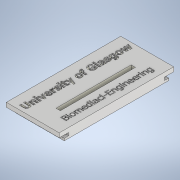
# Autodesk Inventor part: top
Saved by Autodesk Inventor 2021 (Build 250183000, 183)
## iProperties
Created: 2019-01-23
Part Number: top
Material: 常规
Document SubType Name: Modeling
Designer: Guo Xin
Density: 1 g/cm^3
Appearance: 默认
Author: Guo Xin
Autodesk Inventor part; units mm, degrees
(part 1 of 2)
ref_plane "YZ Plane" through (0, 0, 0) normal (1, 0, 0) x (0, 1, 0)
ref_plane "XZ Plane" through (0, 0, 0) normal (0, 1, 0) x (-1, 0, 0)
ref_plane "XY Plane" through (0, 0, 0) normal (0, 0, 1) x (1, 0, 0)
sketch "草图1" plane through (0, 0, 0) normal (0, 1, 0) x (-1, 0, 0)
  line L0 (0, 0) -> (37, 0)
  line L1 (37, 0) -> (37, -80)
  line L2 (37, -80) -> (0, -80)
  line L3 (0, -80) -> (0, 0)
  dimension "d0" = 80
  dimension "d1" = 37
  constraints: 8 end point, 2 parallel, 1 horizontal, 1 perpendicular
  measures "d0" distance between parallel lines of L2 L0
  measures "d1" distance between parallel lines of L3 L1
extrude "拉伸1" add sketch "草图1" along normal mid plane 4
sketch "草图2" plane through (0, -2, 0) normal (1, 0, 0) x (0, 0, -1)
  line L0 (0, 3) -> (6.5, 3)
  line L1 (6.5, 3) -> (6.5, 1)
  line L2 (6.5, 1) -> (0, 1)
  line L3 (0, 1) -> (0, 3)
  line L4 (73.5, 3) -> (80, 3)
  line L5 (80, 3) -> (80, 1)
  line L6 (80, 1) -> (73.5, 1)
  line L7 (73.5, 1) -> (73.5, 3)
  line L8 (0, 2) -> (0, 4) projected
  line L9 (80, 4) -> (80, 0) projected
  line L10 (0, 4) -> (80, 4) projected
  dimension "d4" = 6.5
  dimension "d5" = 1
  dimension "d6" = 2
  dimension "d7" = 6.5
  dimension "d8" = 1
  dimension "d9" = 2
  constraints: 16 end point, 4 parallel, 2 collinear, 2 horizontal, 2 perpendicular, 2 point on line
  measures "d4" distance between parallel lines of L5 L7
  measures "d5" distance between parallel lines of L10 L4
  measures "d6" distance between parallel lines of L4 L6
  measures "d7" distance between parallel lines of L1 L3
  measures "d8" distance between parallel lines of L10 L0
  measures "d9" distance between parallel lines of L2 L0
extrude "拉伸2" cut sketch "草图2" against normal blind 80
sketch "草图3" plane through (0, -1, -6.5) normal (0, 0, 1) x (1, 0, 0)
  line L0 (-37, 2) -> (-31.5, 2)
  line L1 (-31.5, 2) -> (-31.5, 0)
  line L2 (-31.5, 0) -> (-37, 0)
  line L3 (-37, 0) -> (-37, 2)
  line L4 (-37, 0) -> (-37, 2) projected
  line L5 (-37, 2) -> (0, 2) projected
  line L6 (0, 0) -> (-37, 0) projected
  point P0 (0, 1)
  dimension "d12" = 5.5
  constraints: 8 end point, 3 collinear, 2 parallel, 1 horizontal, 1 perpendicular
  measures "d12" distance between parallel lines of L1 L3
extrude "拉伸3" cut sketch "草图3" against normal blind 80
sketch "草图4" plane through (0, -2, 0) normal (1, 0, 0) x (0, 0, -1)
  line L0 (0, 1) -> (3.5, 1)
  line L1 (3.5, 1) -> (3.5, 0)
  line L2 (3.5, 0) -> (0, 0)
  line L3 (0, 0) -> (0, 1)
  line L4 (0, 2) -> (0, 1) projected
  line L5 (6.5, 1) -> (0, 1) projected
  line L6 (80, 0) -> (0, 0) projected
  line L7 (76.5, 1) -> (80, 1)
  line L8 (80, 1) -> (80, 0)
  line L9 (80, 0) -> (76.5, 0)
  line L10 (76.5, 0) -> (76.5, 1)
  line L11 (80, 1) -> (80, 0) projected
  line L12 (80, 1) -> (73.5, 1) projected
  dimension "d15" = 3.5
  dimension "d16" = 3.5
  constraints: 16 end point, 4 collinear, 4 horizontal, 4 parallel, 2 perpendicular, 1 other
  measures "d15" distance between parallel lines of L3 L1
  measures "d16" distance between parallel lines of L8 L10
extrude "拉伸4" cut sketch "草图4" against normal blind 80
sketch "草图8" plane through (0, -2, 0) normal (0, -1, 0) x (1, 0, 0)
  line L0 (-37, -76.5) -> (-34, -76.5)
  line L1 (-34, -76.5) -> (-34, -3.5)
  line L2 (-34, -3.5) -> (-37, -3.5)
  line L3 (-37, -3.5) -> (-37, -76.5)
  line L4 (-37, -3.5) -> (-37, -76.5) projected
  line L5 (-37, -76.5) -> (0, -76.5) projected
  line L6 (0, -3.5) -> (-37, -3.5) projected
  point P0 (0, 0)
  dimension "d29" = 3
  constraints: 8 end point, 3 collinear, 2 parallel, 1 horizontal, 1 perpendicular
  measures "d29" distance between parallel lines of L1 L3
extrude "拉伸6" cut sketch "草图8" against normal blind 1
sketch "草图9" plane through (0, 2, 0) normal (0, 1, 0) x (1, 0, 0)
  line L0 (0, 80) -> (-37, 80)
  line L1 (-37, 80) -> (-37, 0)
  line L2 (-37, 0) -> (0, 0)
  line L3 (0, 0) -> (0, 80)
  line L4 (-37, 0) -> (0, 0) projected
  line L5 (0, 0) -> (0, 80) projected
  line L6 (0, 80) -> (-37, 80) projected
  line L7 (-37, 80) -> (-37, 0) projected
  constraints: 8 end point, 4 collinear, 2 parallel, 1 horizontal, 1 perpendicular
extrude "拉伸7" add sketch "草图9" along normal blind 2
sketch "草图10" plane through (0, -2, 0) normal (0, -1, 0) x (1, 0, 0)
  line L0 (-34, -3.5) -> (0, -3.5)
  line L1 (0, -3.5) -> (0, -76.5)
  line L2 (0, -76.5) -> (-34, -76.5)
  line L3 (-34, -76.5) -> (-34, -3.5)
  line L4 (0, -76.5) -> (0, -3.5) projected
  line L5 (0, -3.5) -> (-34, -3.5) projected
  line L6 (-34, -76.5) -> (0, -76.5) projected
  line L7 (-34, -3.5) -> (-34, -76.5) projected
  point P0 (0, 0)
  constraints: 8 end point, 4 collinear, 2 parallel, 1 horizontal, 1 perpendicular
extrude "拉伸8" add sketch "草图10" along normal blind 0.6
sketch "草图5" plane through (0, 2, 0) normal (0, 1, 0) x (1, 0, 0)
  line L0 (-16, 13.75) -> (-13, 13.75)
  line L1 (-13, 13.75) -> (-13, 66.25)
  line L2 (-13, 66.25) -> (-16, 66.25)
  line L3 (-16, 66.25) -> (-16, 13.75)
  line L4 (-37, 80) -> (-37, 0) projected
  line L5 (-37, 0) -> (0, 0) projected
  dimension "d19" = 21
  dimension "d20" = 3
  dimension "d21" = 52.5
  dimension "d22" = 13.75
  constraints: 8 end point, 2 parallel, 1 horizontal, 1 perpendicular
  measures "d19" distance between parallel lines of L3 L4
  measures "d20" distance between parallel lines of L3 L1
  measures "d21" distance between parallel lines of L2 L0
  measures "d22" distance between parallel lines of L5 L0
extrude "拉伸5" cut sketch "草图5" against normal blind 80 and the other way blind 40
sketch "草图12" plane through (0, 4, 0) normal (0, 1, 0) x (1, 0, 0)
  line L0 (-30.9955, 2.3359) -> (-30.9955, 87.8984) construction
  line L1 (-30.9955, 87.8984) -> (-2.4855, 87.8984) construction
  line L2 (-2.4855, 87.8984) -> (-2.4855, 2.3359) construction
  line L3 (-2.4855, 2.3359) -> (-30.9955, 2.3359) construction
  line L4 (-9.1049, 9.2608) -> (-9.1049, 16.3764) construction
  line L5 (-9.1049, 16.3764) -> (47.4861, 16.3764) construction
  line L6 (47.4861, 16.3764) -> (47.4861, 9.2608) construction
  line L7 (47.4861, 9.2608) -> (-9.1049, 9.2608) construction
  spline S0 degree 2 poles (-25.6349, 4.8765) (-25.6349, 3.8676) (-26.6074, 2.7817) (-27.5474, 2.7817) knots 0 0 0 1 2 2 2
  line L8 (-27.5474, 2.7817) -> (-30.7403, 2.7817)
  line L9 (-30.7403, 2.7817) -> (-30.7403, 4.0377)
  line L10 (-30.7403, 4.0377) -> (-27.6203, 4.0377)
  spline S1 degree 2 poles (-27.6203, 4.0377) (-27.0976, 4.0377) (-26.5871, 4.4308) (-26.5871, 4.8765) knots 0 0 0 1 2 2 2
  spline S2 degree 2 poles (-26.5871, 4.8765) (-26.5871, 5.31) (-27.0774, 5.7152) (-27.6203, 5.7152) knots 0 0 0 1 2 2 2
  line L11 (-27.6203, 5.7152) -> (-30.7403, 5.7152)
  line L12 (-30.7403, 5.7152) -> (-30.7403, 6.9713)
  line L13 (-30.7403, 6.9713) -> (-27.5515, 6.9713)
  spline S3 degree 2 poles (-27.5515, 6.9713) (-26.6276, 6.9713) (-25.6349, 5.9137) (-25.6349, 4.8765) knots 0 0 0 1 2 2 2
  line L14 (-25.7403, 11.3959) -> (-25.7403, 10.2128)
  line L15 (-25.7403, 10.2128) -> (-27.6082, 10.2128)
  spline S4 degree 2 poles (-27.6082, 10.2128) (-27.8391, 10.2128) (-28.2929, 10.1763) (-28.3983, 10.1277) knots 0 0 0 1 2 2 2
  spline S5 degree 2 poles (-28.3983, 10.1277) (-28.5279, 10.0669) (-28.6374, 9.84) (-28.6374, 9.6455) knots 0 0 0 1 2 2 2
  spline S6 degree 2 poles (-28.6374, 9.6455) (-28.6374, 9.5037) (-28.5279, 9.2079) (-28.4104, 9.0418) knots 0 0 0 1 2 2 2
  line L16 (-28.4104, 9.0418) -> (-25.7403, 9.0418)
  line L17 (-25.7403, 9.0418) -> (-25.7403, 7.8667)
  line L18 (-25.7403, 7.8667) -> (-29.5126, 7.8667)
  line L19 (-29.5126, 7.8667) -> (-29.5126, 9.0418)
  line L20 (-29.5126, 9.0418) -> (-29.0952, 9.0418)
  spline S7 degree 2 poles (-29.0952, 9.0418) (-29.3383, 9.3295) (-29.6138, 9.8765) (-29.6138, 10.2087) knots 0 0 0 1 2 2 2
  spline S8 degree 2 poles (-29.6138, 10.2087) (-29.6138, 10.7841) (-28.8845, 11.3959) (-28.1957, 11.3959) knots 0 0 0 1 2 2 2
  line L21 (-28.1957, 11.3959) -> (-25.7403, 11.3959)
  line L22 (-25.7403, 13.4421) -> (-25.7403, 12.2671)
  line L23 (-25.7403, 12.2671) -> (-29.5126, 12.2671)
  line L24 (-29.5126, 12.2671) -> (-29.5126, 13.4421)
  line L25 (-29.5126, 13.4421) -> (-25.7403, 13.4421)
  line L26 (-30.0515, 13.4786) -> (-30.0515, 12.2346)
  line L27 (-30.0515, 12.2346) -> (-30.9672, 12.2346)
  line L28 (-30.9672, 12.2346) -> (-30.9672, 13.4786)
  line L29 (-30.9672, 13.4786) -> (-30.0515, 13.4786)
  line L30 (-29.5126, 17.8708) -> (-25.7403, 16.5175)
  line L31 (-25.7403, 16.5175) -> (-25.7403, 15.233)
  line L32 (-25.7403, 15.233) -> (-29.5126, 13.8919)
  line L33 (-29.5126, 13.8919) -> (-29.5126, 15.1277)
  line L34 (-29.5126, 15.1277) -> (-27.0207, 15.8975)
  line L35 (-27.0207, 15.8975) -> (-29.5126, 16.6593)
  line L36 (-29.5126, 16.6593) -> (-29.5126, 17.8708)
  spline S9 degree 2 poles (-25.639, 20.2533) (-25.639, 19.1836) (-26.66, 18.045) (-27.6041, 18.045) knots 0 0 0 1 2 2 2
  spline S10 degree 2 poles (-27.6041, 18.045) (-28.5279, 18.045) (-29.6301, 19.1066) (-29.6301, 20.0629) knots 0 0 0 1 2 2 2
  spline S11 degree 2 poles (-29.6301, 20.0629) (-29.6301, 20.9259) (-28.6941, 21.8011) (-27.827, 21.8011) knots 0 0 0 1 2 2 2
  line L37 (-27.827, 21.8011) -> (-27.4015, 21.8011)
  line L38 (-27.4015, 21.8011) -> (-27.4015, 19.2201)
  spline S12 degree 2 poles (-27.4015, 19.2201) (-27.1382, 19.2363) (-26.7897, 19.4267) (-26.6844, 19.5807) knots 0 0 0 1 2 2 2
  spline S13 degree 2 poles (-26.6844, 19.5807) (-26.579, 19.7306) (-26.4899, 20.1358) (-26.4899, 20.3748) knots 0 0 0 1 2 2 2
  spline S14 degree 2 poles (-26.4899, 20.3748) (-26.4899, 20.5774) (-26.579, 20.9745) (-26.656, 21.1406) knots 0 0 0 1 2 2 2
  spline S15 degree 2 poles (-26.656, 21.1406) (-26.7168, 21.2865) (-26.8667, 21.5296) (-26.9234, 21.6066) knots 0 0 0 1 2 2 2
  line L39 (-26.9234, 21.6066) -> (-26.9234, 21.7322)
  line L40 (-26.9234, 21.7322) -> (-25.951, 21.7322)
  spline S16 degree 2 poles (-25.951, 21.7322) (-25.8942, 21.5864) (-25.797, 21.3513) (-25.7484, 21.1406) knots 0 0 0 1 2 2 2
  spline S17 degree 2 poles (-25.7484, 21.1406) (-25.6957, 20.9502) (-25.639, 20.545) (-25.639, 20.2533) knots 0 0 0 1 2 2 2
  spline S18 degree 2 poles (-28.1106, 20.6423) (-28.4834, 20.6342) (-28.8764, 20.306) (-28.8764, 19.9697) knots 0 0 0 1 2 2 2
  spline S19 degree 2 poles (-28.8764, 19.9697) (-28.8764, 19.6252) (-28.4631, 19.2363) (-28.1106, 19.216) knots 0 0 0 1 2 2 2
  line L41 (-28.1106, 19.216) -> (-28.1106, 20.6423)
  line L42 (-28.3983, 24.9372) -> (-28.3983, 24.84)
  spline S20 degree 2 poles (-28.3983, 24.84) (-28.4226, 24.7711) (-28.4469, 24.5158) (-28.4469, 24.3619) knots 0 0 0 1 2 2 2
  spline S21 degree 2 poles (-28.4469, 24.3619) (-28.4469, 24.1795) (-28.3375, 23.7703) (-28.2646, 23.5799) knots 0 0 0 1 2 2 2
  line L43 (-28.2646, 23.5799) -> (-25.7403, 23.5799)
  line L44 (-25.7403, 23.5799) -> (-25.7403, 22.4048)
  line L45 (-25.7403, 22.4048) -> (-29.5126, 22.4048)
  line L46 (-29.5126, 22.4048) -> (-29.5126, 23.5799)
  line L47 (-29.5126, 23.5799) -> (-28.9696, 23.5799)
  spline S22 degree 2 poles (-28.9696, 23.5799) (-29.0425, 23.6609) (-29.2694, 23.9445) (-29.3383, 24.062) knots 0 0 0 1 2 2 2
  spline S23 degree 2 poles (-29.3383, 24.062) (-29.4153, 24.1917) (-29.5247, 24.5321) (-29.5247, 24.682) knots 0 0 0 1 2 2 2
  spline S24 degree 2 poles (-29.5247, 24.682) (-29.5247, 24.7387) (-29.5166, 24.8805) (-29.5126, 24.9372) knots 0 0 0 1 2 2 2
  line L48 (-29.5126, 24.9372) -> (-28.3983, 24.9372)
  spline S25 degree 2 poles (-25.639, 26.5337) (-25.639, 26.1204) (-25.8213, 25.3789) (-25.9429, 25.1358) knots 0 0 0 1 2 2 2
  line L49 (-25.9429, 25.1358) -> (-26.9356, 25.1358)
  line L50 (-26.9356, 25.1358) -> (-26.9356, 25.233)
  spline S26 degree 2 poles (-26.9356, 25.233) (-26.8707, 25.3181) (-26.7168, 25.5329) (-26.6317, 25.7233) knots 0 0 0 1 2 2 2
  spline S27 degree 2 poles (-26.6317, 25.7233) (-26.5547, 25.8894) (-26.4453, 26.2987) (-26.4453, 26.5418) knots 0 0 0 1 2 2 2
  spline S28 degree 2 poles (-26.4453, 26.5418) (-26.4453, 26.7889) (-26.5993, 27.1698) (-26.7654, 27.1698) knots 0 0 0 1 2 2 2
  spline S29 degree 2 poles (-26.7654, 27.1698) (-26.895, 27.1698) (-27.0328, 26.9956) (-27.0895, 26.7444) knots 0 0 0 1 2 2 2
  spline S30 degree 2 poles (-27.0895, 26.7444) (-27.126, 26.6107) (-27.203, 26.2014) (-27.2516, 26.0434) knots 0 0 0 1 2 2 2
  spline S31 degree 2 poles (-27.2516, 26.0434) (-27.3894, 25.5977) (-27.9283, 25.152) (-28.3699, 25.152) knots 0 0 0 1 2 2 2
  spline S32 degree 2 poles (-28.3699, 25.152) (-28.6211, 25.152) (-29.0668, 25.3829) (-29.2411, 25.6099) knots 0 0 0 1 2 2 2
  spline S33 degree 2 poles (-29.2411, 25.6099) (-29.4113, 25.8327) (-29.6138, 26.4932) (-29.6138, 26.9105) knots 0 0 0 1 2 2 2
  spline S34 degree 2 poles (-29.6138, 26.9105) (-29.6138, 27.3076) (-29.4558, 27.9721) (-29.3464, 28.199) knots 0 0 0 1 2 2 2
  line L51 (-29.3464, 28.199) -> (-28.3902, 28.199)
  line L52 (-28.3902, 28.199) -> (-28.3902, 28.1058)
  spline S35 degree 2 poles (-28.3902, 28.1058) (-28.4388, 28.045) (-28.5968, 27.7817) (-28.6536, 27.6601) knots 0 0 0 1 2 2 2
  spline S36 degree 2 poles (-28.6536, 27.6601) (-28.7184, 27.5102) (-28.8075, 27.1455) (-28.8075, 26.9551) knots 0 0 0 1 2 2 2
  spline S37 degree 2 poles (-28.8075, 26.9551) (-28.8075, 26.6998) (-28.6333, 26.3473) (-28.4915, 26.3473) knots 0 0 0 1 2 2 2
  spline S38 degree 2 poles (-28.4915, 26.3473) (-28.3618, 26.3473) (-28.216, 26.5215) (-28.143, 26.8133) knots 0 0 0 1 2 2 2
  spline S39 degree 2 poles (-28.143, 26.8133) (-28.1066, 26.9632) (-28.0377, 27.3562) (-27.9769, 27.5385) knots 0 0 0 1 2 2 2
  spline S40 degree 2 poles (-27.9769, 27.5385) (-27.8472, 27.9437) (-27.3408, 28.3651) (-26.9194, 28.3651) knots 0 0 0 1 2 2 2
  spline S41 degree 2 poles (-26.9194, 28.3651) (-26.656, 28.3651) (-26.1738, 28.118) (-26.0117, 27.887) knots 0 0 0 1 2 2 2
  spline S42 degree 2 poles (-26.0117, 27.887) (-25.8335, 27.6479) (-25.639, 26.9915) (-25.639, 26.5337) knots 0 0 0 1 2 2 2
  line L53 (-25.7403, 30.0993) -> (-25.7403, 28.9243)
  line L54 (-25.7403, 28.9243) -> (-29.5126, 28.9243)
  line L55 (-29.5126, 28.9243) -> (-29.5126, 30.0993)
  line L56 (-29.5126, 30.0993) -> (-25.7403, 30.0993)
  line L57 (-30.0515, 30.1358) -> (-30.0515, 28.8919)
  line L58 (-30.0515, 28.8919) -> (-30.9672, 28.8919)
  line L59 (-30.9672, 28.8919) -> (-30.9672, 30.1358)
  line L60 (-30.9672, 30.1358) -> (-30.0515, 30.1358)
  spline S43 degree 2 poles (-25.6673, 32.4413) (-25.6673, 31.7241) (-26.2589, 31.0677) (-26.9315, 31.0677) knots 0 0 0 1 2 2 2
  line L61 (-26.9315, 31.0677) -> (-28.6941, 31.0677)
  line L62 (-28.6941, 31.0677) -> (-28.6941, 30.618)
  line L63 (-28.6941, 30.618) -> (-29.5126, 30.618)
  line L64 (-29.5126, 30.618) -> (-29.5126, 31.0677)
  line L65 (-29.5126, 31.0677) -> (-30.5903, 31.0677)
  line L66 (-30.5903, 31.0677) -> (-30.5903, 32.2428)
  line L67 (-30.5903, 32.2428) -> (-29.5126, 32.2428)
  line L68 (-29.5126, 32.2428) -> (-29.5126, 33.3773)
  line L69 (-29.5126, 33.3773) -> (-28.6941, 33.3773)
  line L70 (-28.6941, 33.3773) -> (-28.6941, 32.2428)
  line L71 (-28.6941, 32.2428) -> (-27.3529, 32.2428)
  spline S44 degree 2 poles (-27.3529, 32.2428) (-27.1544, 32.2428) (-26.8586, 32.2509) (-26.7411, 32.2995) knots 0 0 0 1 2 2 2
  spline S45 degree 2 poles (-26.7411, 32.2995) (-26.6236, 32.3481) (-26.4858, 32.5872) (-26.4858, 32.8141) knots 0 0 0 1 2 2 2
  spline S46 degree 2 poles (-26.4858, 32.8141) (-26.4858, 32.9113) (-26.5668, 33.2152) (-26.5993, 33.276) knots 0 0 0 1 2 2 2
  line L72 (-26.5993, 33.276) -> (-26.5993, 33.3773)
  line L73 (-26.5993, 33.3773) -> (-25.7727, 33.3773)
  spline S47 degree 2 poles (-25.7727, 33.3773) (-25.7241, 33.1868) (-25.6673, 32.7573) (-25.6673, 32.4413) knots 0 0 0 1 2 2 2
  line L74 (-29.5126, 37.3724) -> (-24.3586, 35.4721)
  line L75 (-24.3586, 35.4721) -> (-24.3586, 34.2079)
  line L76 (-24.3586, 34.2079) -> (-25.8335, 34.7792)
  line L77 (-25.8335, 34.7792) -> (-29.5126, 33.3975)
  line L78 (-29.5126, 33.3975) -> (-29.5126, 34.6293)
  line L79 (-29.5126, 34.6293) -> (-27.1463, 35.4235)
  line L80 (-27.1463, 35.4235) -> (-29.5126, 36.165)
  line L81 (-29.5126, 36.165) -> (-29.5126, 37.3724)
  spline S48 degree 2 poles (-27.6244, 43.4462) (-26.6925, 43.4462) (-25.6228, 42.4291) (-25.6228, 41.5013) knots 0 0 0 1 2 2 2
  spline S49 degree 2 poles (-25.6228, 41.5013) (-25.6228, 40.5774) (-26.6925, 39.5523) (-27.6244, 39.5523) knots 0 0 0 1 2 2 2
  spline S50 degree 2 poles (-27.6244, 39.5523) (-28.5644, 39.5523) (-29.6301, 40.5774) (-29.6301, 41.5013) knots 0 0 0 1 2 2 2
  spline S51 degree 2 poles (-29.6301, 41.5013) (-29.6301, 42.4251) (-28.5604, 43.4462) (-27.6244, 43.4462) knots 0 0 0 1 2 2 2
  spline S52 degree 2 poles (-27.6163, 42.2428) (-27.9526, 42.2428) (-28.4023, 42.1334) (-28.5361, 42.0361) knots 0 0 0 1 2 2 2
  spline S53 degree 2 poles (-28.5361, 42.0361) (-28.6779, 41.9308) (-28.7873, 41.6674) (-28.7873, 41.5013) knots 0 0 0 1 2 2 2
  spline S54 degree 2 poles (-28.7873, 41.5013) (-28.7873, 41.3392) (-28.69, 41.0839) (-28.5523, 40.9786) knots 0 0 0 1 2 2 2
  spline S55 degree 2 poles (-28.5523, 40.9786) (-28.4226, 40.8773) (-27.9647, 40.7557) (-27.6163, 40.7557) knots 0 0 0 1 2 2 2
  spline S56 degree 2 poles (-27.6163, 40.7557) (-27.2719, 40.7557) (-26.8464, 40.8692) (-26.7168, 40.9624) knots 0 0 0 1 2 2 2
  spline S57 degree 2 poles (-26.7168, 40.9624) (-26.5871, 41.0556) (-26.4656, 41.3392) (-26.4656, 41.5094) knots 0 0 0 1 2 2 2
  spline S58 degree 2 poles (-26.4656, 41.5094) (-26.4656, 41.6512) (-26.5871, 41.9429) (-26.7087, 42.0321) knots 0 0 0 1 2 2 2
  spline S59 degree 2 poles (-26.7087, 42.0321) (-26.8505, 42.1334) (-27.2597, 42.2428) (-27.6163, 42.2428) knots 0 0 0 1 2 2 2
  line L82 (-30.0758, 46.481) -> (-30.0758, 46.3919)
  spline S60 degree 2 poles (-30.0758, 46.3919) (-30.096, 46.323) (-30.1609, 46.0353) (-30.1609, 45.9097) knots 0 0 0 1 2 2 2
  spline S61 degree 2 poles (-30.1609, 45.9097) (-30.1609, 45.5531) (-29.9015, 45.2938) (-29.5409, 45.2938) knots 0 0 0 1 2 2 2
  line L83 (-29.5409, 45.2938) -> (-29.5126, 45.2938)
  line L84 (-29.5126, 45.2938) -> (-29.5126, 46.2298)
  line L85 (-29.5126, 46.2298) -> (-28.6941, 46.2298)
  line L86 (-28.6941, 46.2298) -> (-28.6941, 45.3343)
  line L87 (-28.6941, 45.3343) -> (-25.7403, 45.3343)
  line L88 (-25.7403, 45.3343) -> (-25.7403, 44.1593)
  line L89 (-25.7403, 44.1593) -> (-28.6941, 44.1593)
  line L90 (-28.6941, 44.1593) -> (-28.6941, 43.6893)
  line L91 (-28.6941, 43.6893) -> (-29.5126, 43.6893)
  line L92 (-29.5126, 43.6893) -> (-29.5126, 44.1593)
  line L93 (-29.5126, 44.1593) -> (-29.6179, 44.1593)
  spline S62 degree 2 poles (-29.6179, 44.1593) (-30.3067, 44.1593) (-30.9955, 44.8846) (-30.9955, 45.622) knots 0 0 0 1 2 2 2
  spline S63 degree 2 poles (-30.9955, 45.622) (-30.9955, 45.8773) (-30.9591, 46.3189) (-30.9267, 46.481) knots 0 0 0 1 2 2 2
  line L94 (-30.9267, 46.481) -> (-30.0758, 46.481)
  spline S64 degree 2 poles (-26.0239, 52.9559) (-25.8902, 52.6277) (-25.6349, 51.5782) (-25.6349, 51.0677) knots 0 0 0 1 2 2 2
  spline S65 degree 2 poles (-25.6349, 51.0677) (-25.6349, 49.8886) (-26.9963, 48.4907) (-28.2443, 48.4907) knots 0 0 0 1 2 2 2
  spline S66 degree 2 poles (-28.2443, 48.4907) (-29.4194, 48.4907) (-30.8375, 49.8886) (-30.8375, 51.1042) knots 0 0 0 1 2 2 2
  spline S67 degree 2 poles (-30.8375, 51.1042) (-30.8375, 51.7322) (-30.5985, 52.5183) (-30.3959, 52.9356) knots 0 0 0 1 2 2 2
  line L95 (-30.3959, 52.9356) -> (-29.2208, 52.9356)
  line L96 (-29.2208, 52.9356) -> (-29.2208, 52.8222)
  spline S68 degree 2 poles (-29.2208, 52.8222) (-29.2897, 52.733) (-29.5531, 52.3927) (-29.6422, 52.2306) knots 0 0 0 1 2 2 2
  spline S69 degree 2 poles (-29.6422, 52.2306) (-29.7516, 52.0442) (-29.9056, 51.5499) (-29.9056, 51.2744) knots 0 0 0 1 2 2 2
  spline S70 degree 2 poles (-29.9056, 51.2744) (-29.9056, 50.9543) (-29.703, 50.4235) (-29.4963, 50.2168) knots 0 0 0 1 2 2 2
  spline S71 degree 2 poles (-29.4963, 50.2168) (-29.2938, 50.0183) (-28.6738, 49.7873) (-28.2646, 49.7873) knots 0 0 0 1 2 2 2
  spline S72 degree 2 poles (-28.2646, 49.7873) (-27.3894, 49.7873) (-26.5547, 50.6666) (-26.5547, 51.4243) knots 0 0 0 1 2 2 2
  spline S73 degree 2 poles (-26.5547, 51.4243) (-26.5547, 51.4932) (-26.5628, 51.6714) (-26.5668, 51.7403) knots 0 0 0 1 2 2 2
  line L97 (-26.5668, 51.7403) -> (-27.5515, 51.7403)
  line L98 (-27.5515, 51.7403) -> (-27.5515, 50.7719)
  line L99 (-27.5515, 50.7719) -> (-28.4874, 50.7719)
  line L100 (-28.4874, 50.7719) -> (-28.4874, 52.9559)
  line L101 (-28.4874, 52.9559) -> (-26.0239, 52.9559)
  line L102 (-25.7403, 55.0102) -> (-25.7403, 53.8351)
  line L103 (-25.7403, 53.8351) -> (-30.9631, 53.8351)
  line L104 (-30.9631, 53.8351) -> (-30.9631, 55.0102)
  line L105 (-30.9631, 55.0102) -> (-25.7403, 55.0102)
  spline S74 degree 2 poles (-26.1414, 57.9883) (-26.0401, 57.8667) (-25.878, 57.6763) (-25.797, 57.5142) knots 0 0 0 1 2 2 2
  spline S75 degree 2 poles (-25.797, 57.5142) (-25.72, 57.3562) (-25.639, 57.0564) (-25.639, 56.7889) knots 0 0 0 1 2 2 2
  spline S76 degree 2 poles (-25.639, 56.7889) (-25.639, 56.2865) (-26.3116, 55.6261) (-26.8221, 55.6261) knots 0 0 0 1 2 2 2
  spline S77 degree 2 poles (-26.8221, 55.6261) (-27.2395, 55.6261) (-27.7581, 55.9624) (-27.908, 56.2784) knots 0 0 0 1 2 2 2
  spline S78 degree 2 poles (-27.908, 56.2784) (-28.062, 56.5985) (-28.1835, 57.4859) (-28.216, 57.9964) knots 0 0 0 1 2 2 2
  line L106 (-28.216, 57.9964) -> (-28.2362, 57.9964)
  spline S79 degree 2 poles (-28.2362, 57.9964) (-28.5482, 57.9964) (-28.7873, 57.5345) (-28.7873, 57.0726) knots 0 0 0 1 2 2 2
  spline S80 degree 2 poles (-28.7873, 57.0726) (-28.7873, 56.8659) (-28.6374, 56.3068) (-28.5198, 56.0434) knots 0 0 0 1 2 2 2
  line L107 (-28.5198, 56.0434) -> (-28.5198, 55.9421)
  line L108 (-28.5198, 55.9421) -> (-29.4315, 55.9421)
  spline S81 degree 2 poles (-29.4315, 55.9421) (-29.4801, 56.1163) (-29.6179, 56.8943) (-29.6179, 57.2914) knots 0 0 0 1 2 2 2
  spline S82 degree 2 poles (-29.6179, 57.2914) (-29.6179, 58.2638) (-28.9696, 59.1552) (-28.3051, 59.1552) knots 0 0 0 1 2 2 2
  line L109 (-28.3051, 59.1552) -> (-25.7403, 59.1552)
  line L110 (-25.7403, 59.1552) -> (-25.7403, 57.9883)
  line L111 (-25.7403, 57.9883) -> (-26.1414, 57.9883)
  line L112 (-26.7249, 57.9883) -> (-27.5069, 57.9883)
  spline S83 degree 2 poles (-27.5069, 57.9883) (-27.4785, 57.6885) (-27.4339, 57.3197) (-27.3691, 57.1415) knots 0 0 0 1 2 2 2
  spline S84 degree 2 poles (-27.3691, 57.1415) (-27.3164, 56.9834) (-27.0976, 56.8133) (-26.9194, 56.8133) knots 0 0 0 1 2 2 2
  spline S85 degree 2 poles (-26.9194, 56.8133) (-26.656, 56.8133) (-26.4574, 57.1009) (-26.4574, 57.3805) knots 0 0 0 1 2 2 2
  spline S86 degree 2 poles (-26.4574, 57.3805) (-26.4574, 57.5345) (-26.5993, 57.8586) (-26.7249, 57.9883) knots 0 0 0 1 2 2 2
  spline S87 degree 2 poles (-25.639, 61.1731) (-25.639, 60.7598) (-25.8213, 60.0183) (-25.9429, 59.7752) knots 0 0 0 1 2 2 2
  line L113 (-25.9429, 59.7752) -> (-26.9356, 59.7752)
  line L114 (-26.9356, 59.7752) -> (-26.9356, 59.8724)
  spline S88 degree 2 poles (-26.9356, 59.8724) (-26.8707, 59.9575) (-26.7168, 60.1723) (-26.6317, 60.3627) knots 0 0 0 1 2 2 2
  spline S89 degree 2 poles (-26.6317, 60.3627) (-26.5547, 60.5288) (-26.4453, 60.9381) (-26.4453, 61.1812) knots 0 0 0 1 2 2 2
  spline S90 degree 2 poles (-26.4453, 61.1812) (-26.4453, 61.4283) (-26.5993, 61.8092) (-26.7654, 61.8092) knots 0 0 0 1 2 2 2
  spline S91 degree 2 poles (-26.7654, 61.8092) (-26.895, 61.8092) (-27.0328, 61.635) (-27.0895, 61.3838) knots 0 0 0 1 2 2 2
  spline S92 degree 2 poles (-27.0895, 61.3838) (-27.126, 61.25) (-27.203, 60.8408) (-27.2516, 60.6828) knots 0 0 0 1 2 2 2
  spline S93 degree 2 poles (-27.2516, 60.6828) (-27.3894, 60.2371) (-27.9283, 59.7914) (-28.3699, 59.7914) knots 0 0 0 1 2 2 2
  spline S94 degree 2 poles (-28.3699, 59.7914) (-28.6211, 59.7914) (-29.0668, 60.0223) (-29.2411, 60.2492) knots 0 0 0 1 2 2 2
  spline S95 degree 2 poles (-29.2411, 60.2492) (-29.4113, 60.4721) (-29.6138, 61.1325) (-29.6138, 61.5499) knots 0 0 0 1 2 2 2
  spline S96 degree 2 poles (-29.6138, 61.5499) (-29.6138, 61.947) (-29.4558, 62.6115) (-29.3464, 62.8384) knots 0 0 0 1 2 2 2
  line L115 (-29.3464, 62.8384) -> (-28.3902, 62.8384)
  line L116 (-28.3902, 62.8384) -> (-28.3902, 62.7452)
  spline S97 degree 2 poles (-28.3902, 62.7452) (-28.4388, 62.6844) (-28.5968, 62.421) (-28.6536, 62.2995) knots 0 0 0 1 2 2 2
  spline S98 degree 2 poles (-28.6536, 62.2995) (-28.7184, 62.1496) (-28.8075, 61.7849) (-28.8075, 61.5945) knots 0 0 0 1 2 2 2
  spline S99 degree 2 poles (-28.8075, 61.5945) (-28.8075, 61.3392) (-28.6333, 60.9867) (-28.4915, 60.9867) knots 0 0 0 1 2 2 2
  spline S100 degree 2 poles (-28.4915, 60.9867) (-28.3618, 60.9867) (-28.216, 61.1609) (-28.143, 61.4526) knots 0 0 0 1 2 2 2
  spline S101 degree 2 poles (-28.143, 61.4526) (-28.1066, 61.6026) (-28.0377, 61.9956) (-27.9769, 62.1779) knots 0 0 0 1 2 2 2
  spline S102 degree 2 poles (-27.9769, 62.1779) (-27.8472, 62.5831) (-27.3408, 63.0045) (-26.9194, 63.0045) knots 0 0 0 1 2 2 2
  spline S103 degree 2 poles (-26.9194, 63.0045) (-26.656, 63.0045) (-26.1738, 62.7573) (-26.0117, 62.5264) knots 0 0 0 1 2 2 2
  spline S104 degree 2 poles (-26.0117, 62.5264) (-25.8335, 62.2873) (-25.639, 61.6309) (-25.639, 61.1731) knots 0 0 0 1 2 2 2
  spline S105 degree 2 poles (-26.1738, 66.9915) (-25.6511, 66.9915) (-24.9177, 66.6876) (-24.7151, 66.4283) knots 0 0 0 1 2 2 2
  spline S106 degree 2 poles (-24.7151, 66.4283) (-24.5085, 66.165) (-24.3221, 65.4356) (-24.3221, 64.9899) knots 0 0 0 1 2 2 2
  spline S107 degree 2 poles (-24.3221, 64.9899) (-24.3221, 64.6131) (-24.4194, 63.9364) (-24.4842, 63.6893) knots 0 0 0 1 2 2 2
  line L117 (-24.4842, 63.6893) -> (-25.4283, 63.6893)
  line L118 (-25.4283, 63.6893) -> (-25.4283, 63.827)
  spline S108 degree 2 poles (-25.4283, 63.827) (-25.3959, 63.9121) (-25.3148, 64.1512) (-25.2824, 64.2727) knots 0 0 0 1 2 2 2
  spline S109 degree 2 poles (-25.2824, 64.2727) (-25.2459, 64.4186) (-25.1973, 64.6941) (-25.1973, 64.8359) knots 0 0 0 1 2 2 2
  spline S110 degree 2 poles (-25.1973, 64.8359) (-25.1973, 65.1358) (-25.3189, 65.5329) (-25.4323, 65.6342) knots 0 0 0 1 2 2 2
  spline S111 degree 2 poles (-25.4323, 65.6342) (-25.5498, 65.7355) (-25.8659, 65.8165) (-26.109, 65.8165) knots 0 0 0 1 2 2 2
  line L119 (-26.109, 65.8165) -> (-26.1779, 65.8165)
  spline S112 degree 2 poles (-26.1779, 65.8165) (-26.0036, 65.618) (-25.7929, 65.0993) (-25.7929, 64.8238) knots 0 0 0 1 2 2 2
  spline S113 degree 2 poles (-25.7929, 64.8238) (-25.7929, 64.0904) (-26.7451, 63.2962) (-27.7216, 63.2962) knots 0 0 0 1 2 2 2
  spline S114 degree 2 poles (-27.7216, 63.2962) (-28.1633, 63.2962) (-28.8683, 63.5393) (-29.1155, 63.7582) knots 0 0 0 1 2 2 2
  spline S115 degree 2 poles (-29.1155, 63.7582) (-29.3545, 63.9688) (-29.6138, 64.5564) (-29.6138, 64.8765) knots 0 0 0 1 2 2 2
  spline S116 degree 2 poles (-29.6138, 64.8765) (-29.6138, 65.1641) (-29.468, 65.622) (-29.3464, 65.8084) knots 0 0 0 1 2 2 2
  line L120 (-29.3464, 65.8084) -> (-29.5126, 65.853)
  line L121 (-29.5126, 65.853) -> (-29.5126, 66.9915)
  line L122 (-29.5126, 66.9915) -> (-26.1738, 66.9915)
  line L123 (-26.9275, 65.8165) -> (-28.6374, 65.8165)
  spline S117 degree 2 poles (-28.6374, 65.8165) (-28.6779, 65.7314) (-28.7305, 65.4761) (-28.7305, 65.3465) knots 0 0 0 1 2 2 2
  spline S118 degree 2 poles (-28.7305, 65.3465) (-28.7305, 64.9251) (-28.1835, 64.4996) (-27.6933, 64.4996) knots 0 0 0 1 2 2 2
  spline S119 degree 2 poles (-27.6933, 64.4996) (-27.4502, 64.4996) (-27.1098, 64.5645) (-26.9801, 64.6496) knots 0 0 0 1 2 2 2
  spline S120 degree 2 poles (-26.9801, 64.6496) (-26.8505, 64.7346) (-26.7208, 65.0061) (-26.7208, 65.2168) knots 0 0 0 1 2 2 2
  spline S121 degree 2 poles (-26.7208, 65.2168) (-26.7208, 65.3748) (-26.8302, 65.6787) (-26.9275, 65.8165) knots 0 0 0 1 2 2 2
  spline S122 degree 2 poles (-27.6244, 71.5094) (-26.6925, 71.5094) (-25.6228, 70.4923) (-25.6228, 69.5645) knots 0 0 0 1 2 2 2
  spline S123 degree 2 poles (-25.6228, 69.5645) (-25.6228, 68.6406) (-26.6925, 67.6155) (-27.6244, 67.6155) knots 0 0 0 1 2 2 2
  spline S124 degree 2 poles (-27.6244, 67.6155) (-28.5644, 67.6155) (-29.6301, 68.6406) (-29.6301, 69.5645) knots 0 0 0 1 2 2 2
  spline S125 degree 2 poles (-29.6301, 69.5645) (-29.6301, 70.4883) (-28.5604, 71.5094) (-27.6244, 71.5094) knots 0 0 0 1 2 2 2
  spline S126 degree 2 poles (-27.6163, 70.306) (-27.9526, 70.306) (-28.4023, 70.1966) (-28.5361, 70.0993) knots 0 0 0 1 2 2 2
  spline S127 degree 2 poles (-28.5361, 70.0993) (-28.6779, 69.994) (-28.7873, 69.7306) (-28.7873, 69.5645) knots 0 0 0 1 2 2 2
  spline S128 degree 2 poles (-28.7873, 69.5645) (-28.7873, 69.4024) (-28.69, 69.1471) (-28.5523, 69.0418) knots 0 0 0 1 2 2 2
  spline S129 degree 2 poles (-28.5523, 69.0418) (-28.4226, 68.9405) (-27.9647, 68.8189) (-27.6163, 68.8189) knots 0 0 0 1 2 2 2
  spline S130 degree 2 poles (-27.6163, 68.8189) (-27.2719, 68.8189) (-26.8464, 68.9324) (-26.7168, 69.0256) knots 0 0 0 1 2 2 2
  spline S131 degree 2 poles (-26.7168, 69.0256) (-26.5871, 69.1188) (-26.4656, 69.4024) (-26.4656, 69.5726) knots 0 0 0 1 2 2 2
  spline S132 degree 2 poles (-26.4656, 69.5726) (-26.4656, 69.7144) (-26.5871, 70.0061) (-26.7087, 70.0953) knots 0 0 0 1 2 2 2
  spline S133 degree 2 poles (-26.7087, 70.0953) (-26.8505, 70.1966) (-27.2597, 70.306) (-27.6163, 70.306) knots 0 0 0 1 2 2 2
  line L124 (-29.5126, 77.7533) -> (-25.7403, 76.6512)
  line L125 (-25.7403, 76.6512) -> (-25.7403, 75.4032)
  line L126 (-25.7403, 75.4032) -> (-28.1795, 74.7387)
  line L127 (-28.1795, 74.7387) -> (-25.7403, 74.0742)
  line L128 (-25.7403, 74.0742) -> (-25.7403, 72.8262)
  line L129 (-25.7403, 72.8262) -> (-29.5126, 71.7322)
  line L130 (-29.5126, 71.7322) -> (-29.5126, 72.968)
  line L131 (-29.5126, 72.968) -> (-27.0166, 73.5475)
  line L132 (-27.0166, 73.5475) -> (-29.5126, 74.2606)
  line L133 (-29.5126, 74.2606) -> (-29.5126, 75.3019)
  line L134 (-29.5126, 75.3019) -> (-27.0166, 75.9745)
  line L135 (-27.0166, 75.9745) -> (-29.5126, 76.5458)
  line L136 (-29.5126, 76.5458) -> (-29.5126, 77.7533)
  spline S134 degree 2 poles (-6.1551, 12.6903) (-5.8569, 12.6903) (-5.3999, 12.4407) (-5.2507, 12.2332) knots 0 0 0 1 2 2 2
  spline S135 degree 2 poles (-5.2507, 12.2332) (-5.0757, 11.9836) (-4.9266, 11.4164) (-4.9266, 10.9691) knots 0 0 0 1 2 2 2
  line L137 (-4.9266, 10.9691) -> (-4.9266, 9.7081)
  line L138 (-4.9266, 9.7081) -> (-8.9266, 9.7081)
  line L139 (-8.9266, 9.7081) -> (-8.9266, 10.8751)
  spline S136 degree 2 poles (-8.9266, 10.8751) (-8.9266, 11.3451) (-8.8715, 11.8118) (-8.7645, 12.029) knots 0 0 0 1 2 2 2
  spline S137 degree 2 poles (-8.7645, 12.029) (-8.6511, 12.2657) (-8.2783, 12.4828) (-8.0255, 12.4828) knots 0 0 0 1 2 2 2
  spline S138 degree 2 poles (-8.0255, 12.4828) (-7.7434, 12.4828) (-7.2961, 12.1554) (-7.1697, 11.8669) knots 0 0 0 1 2 2 2
  line L140 (-7.1697, 11.8669) -> (-7.1503, 11.8669)
  spline S139 degree 2 poles (-7.1503, 11.8669) (-7.053, 12.2592) (-6.5376, 12.6903) (-6.1551, 12.6903) knots 0 0 0 1 2 2 2
  spline S140 degree 2 poles (-6.1324, 12.0809) (-6.3593, 12.0809) (-6.6511, 11.9383) (-6.7548, 11.7243) knots 0 0 0 1 2 2 2
  spline S141 degree 2 poles (-6.7548, 11.7243) (-6.8196, 11.5849) (-6.8585, 11.2575) (-6.8585, 10.9561) knots 0 0 0 1 2 2 2
  line L141 (-6.8585, 10.9561) -> (-6.8585, 10.2916)
  line L142 (-6.8585, 10.2916) -> (-5.3804, 10.2916)
  line L143 (-5.3804, 10.2916) -> (-5.3804, 10.7681)
  spline S142 degree 2 poles (-5.3804, 10.7681) (-5.3804, 11.1506) (-5.4452, 11.5947) (-5.549, 11.7632) knots 0 0 0 1 2 2 2
  spline S143 degree 2 poles (-5.549, 11.7632) (-5.6559, 11.9285) (-5.9217, 12.0809) (-6.1324, 12.0809) knots 0 0 0 1 2 2 2
  spline S144 degree 2 poles (-7.9509, 11.8734) (-8.0935, 11.8734) (-8.3075, 11.7665) (-8.3691, 11.6498) knots 0 0 0 1 2 2 2
  spline S145 degree 2 poles (-8.3691, 11.6498) (-8.4404, 11.5071) (-8.4728, 11.1603) (-8.4728, 10.8524) knots 0 0 0 1 2 2 2
  line L144 (-8.4728, 10.8524) -> (-8.4728, 10.2916)
  line L145 (-8.4728, 10.2916) -> (-7.3026, 10.2916)
  line L146 (-7.3026, 10.2916) -> (-7.3026, 10.9561)
  spline S146 degree 2 poles (-7.3026, 10.9561) (-7.3026, 11.2316) (-7.3545, 11.4909) (-7.4355, 11.6271) knots 0 0 0 1 2 2 2
  spline S147 degree 2 poles (-7.4355, 11.6271) (-7.5133, 11.76) (-7.7629, 11.8734) (-7.9509, 11.8734) knots 0 0 0 1 2 2 2
  line L147 (-4.9266, 13.7924) -> (-4.9266, 13.2381)
  line L148 (-4.9266, 13.2381) -> (-7.9282, 13.2381)
  line L149 (-7.9282, 13.2381) -> (-7.9282, 13.7924)
  line L150 (-7.9282, 13.7924) -> (-4.9266, 13.7924)
  line L151 (-8.4274, 13.8345) -> (-8.4274, 13.2024)
  line L152 (-8.4274, 13.2024) -> (-8.9525, 13.2024)
  line L153 (-8.9525, 13.2024) -> (-8.9525, 13.8345)
  line L154 (-8.9525, 13.8345) -> (-8.4274, 13.8345)
  spline S148 degree 2 poles (-6.4274, 17.3224) (-5.6689, 17.3224) (-4.8423, 16.5185) (-4.8423, 15.8507) knots 0 0 0 1 2 2 2
  spline S149 degree 2 poles (-4.8423, 15.8507) (-4.8423, 15.1635) (-5.6948, 14.3759) (-6.4274, 14.3759) knots 0 0 0 1 2 2 2
  spline S150 degree 2 poles (-6.4274, 14.3759) (-7.1794, 14.3759) (-8.0125, 15.1862) (-8.0125, 15.8507) knots 0 0 0 1 2 2 2
  spline S151 degree 2 poles (-8.0125, 15.8507) (-8.0125, 16.5185) (-7.1827, 17.3224) (-6.4274, 17.3224) knots 0 0 0 1 2 2 2
  spline S152 degree 2 poles (-6.4274, 16.7486) (-7.0109, 16.7486) (-7.5781, 16.2819) (-7.5781, 15.8507) knots 0 0 0 1 2 2 2
  spline S153 degree 2 poles (-7.5781, 15.8507) (-7.5781, 15.4196) (-7.0109, 14.9496) (-6.4274, 14.9496) knots 0 0 0 1 2 2 2
  spline S154 degree 2 poles (-6.4274, 14.9496) (-5.8601, 14.9496) (-5.2767, 15.4196) (-5.2767, 15.8507) knots 0 0 0 1 2 2 2
  spline S155 degree 2 poles (-5.2767, 15.8507) (-5.2767, 16.2786) (-5.8504, 16.7486) (-6.4274, 16.7486) knots 0 0 0 1 2 2 2
  line L155 (-4.9266, 21.64) -> (-6.664, 21.64)
  spline S156 degree 2 poles (-6.664, 21.64) (-6.8715, 21.64) (-7.2248, 21.6044) (-7.3221, 21.5493) knots 0 0 0 1 2 2 2
  spline S157 degree 2 poles (-7.3221, 21.5493) (-7.429, 21.4877) (-7.5328, 21.2705) (-7.5328, 21.0825) knots 0 0 0 1 2 2 2
  spline S158 degree 2 poles (-7.5328, 21.0825) (-7.5328, 20.914) (-7.3415, 20.5185) (-7.16, 20.3078) knots 0 0 0 1 2 2 2
  spline S159 degree 2 poles (-7.16, 20.3078) (-7.1146, 20.311) (-6.9882, 20.3208) (-6.9039, 20.3208) knots 0 0 0 1 2 2 2
  line L156 (-6.9039, 20.3208) -> (-4.9266, 20.3208)
  line L157 (-4.9266, 20.3208) -> (-4.9266, 19.7665)
  line L158 (-4.9266, 19.7665) -> (-6.664, 19.7665)
  spline S160 degree 2 poles (-6.664, 19.7665) (-6.8715, 19.7665) (-7.2248, 19.7308) (-7.3221, 19.6757) knots 0 0 0 1 2 2 2
  spline S161 degree 2 poles (-7.3221, 19.6757) (-7.429, 19.6141) (-7.5328, 19.3969) (-7.5328, 19.2089) knots 0 0 0 1 2 2 2
  spline S162 degree 2 poles (-7.5328, 19.2089) (-7.5328, 19.0306) (-7.3285, 18.6319) (-7.1697, 18.4472) knots 0 0 0 1 2 2 2
  line L159 (-7.1697, 18.4472) -> (-4.9266, 18.4472)
  line L160 (-4.9266, 18.4472) -> (-4.9266, 17.8929)
  line L161 (-4.9266, 17.8929) -> (-7.9282, 17.8929)
  line L162 (-7.9282, 17.8929) -> (-7.9282, 18.4472)
  line L163 (-7.9282, 18.4472) -> (-7.5976, 18.4472)
  spline S163 degree 2 poles (-7.5976, 18.4472) (-7.7953, 18.6644) (-8.0125, 19.0955) (-8.0125, 19.3516) knots 0 0 0 1 2 2 2
  spline S164 degree 2 poles (-8.0125, 19.3516) (-8.0125, 19.6433) (-7.7694, 20.0971) (-7.4939, 20.2138) knots 0 0 0 1 2 2 2
  spline S165 degree 2 poles (-7.4939, 20.2138) (-7.7499, 20.4666) (-8.0125, 20.9431) (-8.0125, 21.2251) knots 0 0 0 1 2 2 2
  spline S166 degree 2 poles (-8.0125, 21.2251) (-8.0125, 21.4391) (-7.8926, 21.7859) (-7.7564, 21.9156) knots 0 0 0 1 2 2 2
  spline S167 degree 2 poles (-7.7564, 21.9156) (-7.6203, 22.0485) (-7.2118, 22.1943) (-6.9039, 22.1943) knots 0 0 0 1 2 2 2
  line L164 (-6.9039, 22.1943) -> (-4.9266, 22.1943)
  line L165 (-4.9266, 22.1943) -> (-4.9266, 21.64)
  spline S168 degree 2 poles (-4.8585, 24.405) (-4.8585, 23.6174) (-5.6657, 22.7454) (-6.4112, 22.7454) knots 0 0 0 1 2 2 2
  spline S169 degree 2 poles (-6.4112, 22.7454) (-7.1438, 22.7454) (-8.0125, 23.5914) (-8.0125, 24.2721) knots 0 0 0 1 2 2 2
  spline S170 degree 2 poles (-8.0125, 24.2721) (-8.0125, 24.5801) (-7.8504, 25.0501) (-7.6786, 25.2284) knots 0 0 0 1 2 2 2
  spline S171 degree 2 poles (-7.6786, 25.2284) (-7.5068, 25.4067) (-7.0109, 25.5947) (-6.6511, 25.5947) knots 0 0 0 1 2 2 2
  line L166 (-6.6511, 25.5947) -> (-6.3755, 25.5947)
  line L167 (-6.3755, 25.5947) -> (-6.3755, 23.3094)
  spline S172 degree 2 poles (-6.3755, 23.3094) (-5.8537, 23.3094) (-5.2994, 23.8896) (-5.2994, 24.3986) knots 0 0 0 1 2 2 2
  spline S173 degree 2 poles (-5.2994, 24.3986) (-5.2994, 24.5833) (-5.3739, 24.9334) (-5.4323, 25.076) knots 0 0 0 1 2 2 2
  spline S174 degree 2 poles (-5.4323, 25.076) (-5.4971, 25.2251) (-5.6105, 25.4326) (-5.6624, 25.5007) knots 0 0 0 1 2 2 2
  line L168 (-5.6624, 25.5007) -> (-5.6624, 25.5331)
  line L169 (-5.6624, 25.5331) -> (-5.1114, 25.5331)
  spline S175 degree 2 poles (-5.1114, 25.5331) (-5.0757, 25.4358) (-4.972, 25.1473) (-4.9428, 25.0306) knots 0 0 0 1 2 2 2
  spline S176 degree 2 poles (-4.9428, 25.0306) (-4.9007, 24.8686) (-4.8585, 24.606) (-4.8585, 24.405) knots 0 0 0 1 2 2 2
  spline S177 degree 2 poles (-6.7613, 25.0533) (-6.9655, 25.0469) (-7.2637, 24.9528) (-7.3642, 24.8653) knots 0 0 0 1 2 2 2
  spline S178 degree 2 poles (-7.3642, 24.8653) (-7.4776, 24.7681) (-7.5976, 24.4634) (-7.5976, 24.2397) knots 0 0 0 1 2 2 2
  spline S179 degree 2 poles (-7.5976, 24.2397) (-7.5976, 24.0161) (-7.4776, 23.7081) (-7.361, 23.5817) knots 0 0 0 1 2 2 2
  spline S180 degree 2 poles (-7.361, 23.5817) (-7.241, 23.4585) (-6.9525, 23.3256) (-6.7613, 23.3094) knots 0 0 0 1 2 2 2
  line L170 (-6.7613, 23.3094) -> (-6.7613, 25.0533)
  line L171 (-4.9266, 28.6935) -> (-4.9266, 28.1392)
  line L172 (-4.9266, 28.1392) -> (-5.2313, 28.1392)
  spline S181 degree 2 poles (-5.2313, 28.1392) (-5.134, 28.0096) (-5.0044, 27.8216) (-4.9493, 27.6952) knots 0 0 0 1 2 2 2
  spline S182 degree 2 poles (-4.9493, 27.6952) (-4.8974, 27.5752) (-4.8423, 27.3224) (-4.8423, 27.1538) knots 0 0 0 1 2 2 2
  spline S183 degree 2 poles (-4.8423, 27.1538) (-4.8423, 26.8848) (-5.0465, 26.4277) (-5.2443, 26.2689) knots 0 0 0 1 2 2 2
  spline S184 degree 2 poles (-5.2443, 26.2689) (-5.442, 26.1068) (-6.0255, 25.9285) (-6.4047, 25.9285) knots 0 0 0 1 2 2 2
  spline S185 degree 2 poles (-6.4047, 25.9285) (-6.8002, 25.9285) (-7.3772, 26.1522) (-7.5943, 26.3499) knots 0 0 0 1 2 2 2
  spline S186 degree 2 poles (-7.5943, 26.3499) (-7.7888, 26.5315) (-8.0125, 27.0404) (-8.0125, 27.3224) knots 0 0 0 1 2 2 2
  spline S187 degree 2 poles (-8.0125, 27.3224) (-8.0125, 27.5687) (-7.912, 27.935) (-7.8083, 28.1392) knots 0 0 0 1 2 2 2
  line L173 (-7.8083, 28.1392) -> (-9.1049, 28.1392)
  line L174 (-9.1049, 28.1392) -> (-9.1049, 28.6935)
  line L175 (-9.1049, 28.6935) -> (-4.9266, 28.6935)
  line L176 (-5.6559, 28.1392) -> (-7.3901, 28.1392)
  spline S188 degree 2 poles (-7.3901, 28.1392) (-7.4809, 27.9318) (-7.549, 27.6044) (-7.549, 27.4131) knots 0 0 0 1 2 2 2
  spline S189 degree 2 poles (-7.549, 27.4131) (-7.549, 26.9853) (-6.9655, 26.5023) (-6.4144, 26.5023) knots 0 0 0 1 2 2 2
  spline S190 degree 2 poles (-6.4144, 26.5023) (-5.8828, 26.5023) (-5.3221, 26.8751) (-5.3221, 27.2835) knots 0 0 0 1 2 2 2
  spline S191 degree 2 poles (-5.3221, 27.2835) (-5.3221, 27.5007) (-5.5036, 27.9447) (-5.6559, 28.1392) knots 0 0 0 1 2 2 2
  line L177 (-4.9266, 30.0614) -> (-4.9266, 29.5071)
  line L178 (-4.9266, 29.5071) -> (-7.9282, 29.5071)
  line L179 (-7.9282, 29.5071) -> (-7.9282, 30.0614)
  line L180 (-7.9282, 30.0614) -> (-4.9266, 30.0614)
  line L181 (-8.4274, 30.1036) -> (-8.4274, 29.4715)
  line L182 (-8.4274, 29.4715) -> (-8.9525, 29.4715)
  line L183 (-8.9525, 29.4715) -> (-8.9525, 30.1036)
  line L184 (-8.9525, 30.1036) -> (-8.4274, 30.1036)
  spline S192 degree 2 poles (-5.2443, 32.7162) (-5.1989, 32.6481) (-5.0368, 32.4212) (-4.9882, 32.3143) knots 0 0 0 1 2 2 2
  spline S193 degree 2 poles (-4.9882, 32.3143) (-4.9169, 32.1684) (-4.8423, 31.8929) (-4.8423, 31.6465) knots 0 0 0 1 2 2 2
  spline S194 degree 2 poles (-4.8423, 31.6465) (-4.8423, 31.4423) (-4.9817, 31.076) (-5.1081, 30.9366) knots 0 0 0 1 2 2 2
  spline S195 degree 2 poles (-5.1081, 30.9366) (-5.2313, 30.8037) (-5.5943, 30.6449) (-5.7953, 30.6449) knots 0 0 0 1 2 2 2
  spline S196 degree 2 poles (-5.7953, 30.6449) (-6.1065, 30.6449) (-6.5473, 30.9334) (-6.6738, 31.2478) knots 0 0 0 1 2 2 2
  spline S197 degree 2 poles (-6.6738, 31.2478) (-6.7905, 31.5234) (-6.878, 32.2786) (-6.9007, 32.7162) knots 0 0 0 1 2 2 2
  line L185 (-6.9007, 32.7162) -> (-6.9979, 32.7162)
  spline S198 degree 2 poles (-6.9979, 32.7162) (-7.1729, 32.7162) (-7.3901, 32.5995) (-7.4517, 32.4926) knots 0 0 0 1 2 2 2
  spline S199 degree 2 poles (-7.4517, 32.4926) (-7.5133, 32.3856) (-7.5522, 32.0776) (-7.5522, 31.9156) knots 0 0 0 1 2 2 2
  spline S200 degree 2 poles (-7.5522, 31.9156) (-7.5522, 31.7243) (-7.4485, 31.2057) (-7.348, 30.9464) knots 0 0 0 1 2 2 2
  line L186 (-7.348, 30.9464) -> (-7.348, 30.914)
  line L187 (-7.348, 30.914) -> (-7.8634, 30.914)
  spline S201 degree 2 poles (-7.8634, 30.914) (-7.9023, 31.0663) (-7.9995, 31.64) (-7.9995, 31.9221) knots 0 0 0 1 2 2 2
  spline S202 degree 2 poles (-7.9995, 31.9221) (-7.9995, 32.2592) (-7.9023, 32.7259) (-7.7759, 32.914) knots 0 0 0 1 2 2 2
  spline S203 degree 2 poles (-7.7759, 32.914) (-7.6527, 33.0922) (-7.2605, 33.2705) (-6.9785, 33.2705) knots 0 0 0 1 2 2 2
  line L188 (-6.9785, 33.2705) -> (-4.9266, 33.2705)
  line L189 (-4.9266, 33.2705) -> (-4.9266, 32.7162)
  line L190 (-4.9266, 32.7162) -> (-5.2443, 32.7162)
  line L191 (-5.6657, 32.7162) -> (-6.4987, 32.7162)
  spline S204 degree 2 poles (-6.4987, 32.7162) (-6.4825, 32.5185) (-6.4274, 31.9156) (-6.3755, 31.7276) knots 0 0 0 1 2 2 2
  spline S205 degree 2 poles (-6.3755, 31.7276) (-6.314, 31.5071) (-6.0579, 31.2187) (-5.831, 31.2187) knots 0 0 0 1 2 2 2
  spline S206 degree 2 poles (-5.831, 31.2187) (-5.5717, 31.2187) (-5.3091, 31.5363) (-5.3091, 31.8443) knots 0 0 0 1 2 2 2
  spline S207 degree 2 poles (-5.3091, 31.8443) (-5.3091, 32.1068) (-5.5133, 32.5315) (-5.6657, 32.7162) knots 0 0 0 1 2 2 2
  spline S208 degree 2 poles (-4.8585, 35.3613) (-4.8585, 35.0242) (-5.0498, 34.4569) (-5.2443, 34.2527) knots 0 0 0 1 2 2 2
  spline S209 degree 2 poles (-5.2443, 34.2527) (-5.4355, 34.0485) (-6.0255, 33.8248) (-6.4209, 33.8248) knots 0 0 0 1 2 2 2
  spline S210 degree 2 poles (-6.4209, 33.8248) (-6.8164, 33.8248) (-7.3934, 34.0582) (-7.5879, 34.2527) knots 0 0 0 1 2 2 2
  spline S211 degree 2 poles (-7.5879, 34.2527) (-7.7856, 34.4472) (-7.9963, 35.0306) (-7.9963, 35.3613) knots 0 0 0 1 2 2 2
  spline S212 degree 2 poles (-7.9963, 35.3613) (-7.9963, 35.6336) (-7.8569, 36.1392) (-7.7661, 36.337) knots 0 0 0 1 2 2 2
  line L192 (-7.7661, 36.337) -> (-7.1989, 36.337)
  line L193 (-7.1989, 36.337) -> (-7.1989, 36.3046)
  spline S213 degree 2 poles (-7.1989, 36.3046) (-7.2443, 36.2462) (-7.361, 36.0582) (-7.4225, 35.9253) knots 0 0 0 1 2 2 2
  spline S214 degree 2 poles (-7.4225, 35.9253) (-7.4744, 35.8118) (-7.5554, 35.4974) (-7.5554, 35.3516) knots 0 0 0 1 2 2 2
  spline S215 degree 2 poles (-7.5554, 35.3516) (-7.5554, 34.9204) (-6.9623, 34.3986) (-6.4209, 34.3986) knots 0 0 0 1 2 2 2
  spline S216 degree 2 poles (-6.4209, 34.3986) (-5.8926, 34.3986) (-5.2994, 34.9042) (-5.2994, 35.3516) knots 0 0 0 1 2 2 2
  spline S217 degree 2 poles (-5.2994, 35.3516) (-5.2994, 35.6238) (-5.5036, 36.1165) (-5.6624, 36.3046) knots 0 0 0 1 2 2 2
  line L194 (-5.6624, 36.3046) -> (-5.6624, 36.337)
  line L195 (-5.6624, 36.337) -> (-5.0952, 36.337)
  spline S218 degree 2 poles (-5.0952, 36.337) (-5.0595, 36.2559) (-4.959, 36.0063) (-4.9363, 35.9058) knots 0 0 0 1 2 2 2
  spline S219 degree 2 poles (-4.9363, 35.9058) (-4.8974, 35.7632) (-4.8585, 35.5396) (-4.8585, 35.3613) knots 0 0 0 1 2 2 2
  line L196 (-4.9266, 37.4067) -> (-4.9266, 36.8524)
  line L197 (-4.9266, 36.8524) -> (-9.1049, 36.8524)
  line L198 (-9.1049, 36.8524) -> (-9.1049, 37.4067)
  line L199 (-9.1049, 37.4067) -> (-4.9266, 37.4067)
  line L200 (-6.4339, 39.7535) -> (-6.4339, 38.0874)
  line L201 (-6.4339, 38.0874) -> (-6.9201, 38.0874)
  line L202 (-6.9201, 38.0874) -> (-6.9201, 39.7535)
  line L203 (-6.9201, 39.7535) -> (-6.4339, 39.7535)
  line L204 (-4.9266, 40.4666) -> (-8.9266, 40.4666)
  line L205 (-8.9266, 40.4666) -> (-8.9266, 43.2187)
  line L206 (-8.9266, 43.2187) -> (-8.4533, 43.2187)
  line L207 (-8.4533, 43.2187) -> (-8.4533, 41.0501)
  line L208 (-8.4533, 41.0501) -> (-7.3577, 41.0501)
  line L209 (-7.3577, 41.0501) -> (-7.3577, 43.0695)
  line L210 (-7.3577, 43.0695) -> (-6.8845, 43.0695)
  line L211 (-6.8845, 43.0695) -> (-6.8845, 41.0501)
  line L212 (-6.8845, 41.0501) -> (-5.3999, 41.0501)
  line L213 (-5.3999, 41.0501) -> (-5.3999, 43.2187)
  line L214 (-5.3999, 43.2187) -> (-4.9266, 43.2187)
  line L215 (-4.9266, 43.2187) -> (-4.9266, 40.4666)
  line L216 (-4.9266, 46.4083) -> (-4.9266, 45.854)
  line L217 (-4.9266, 45.854) -> (-6.6381, 45.854)
  spline S220 degree 2 poles (-6.6381, 45.854) (-6.8456, 45.854) (-7.2021, 45.8086) (-7.3091, 45.747) knots 0 0 0 1 2 2 2
  spline S221 degree 2 poles (-7.3091, 45.747) (-7.4225, 45.6789) (-7.5328, 45.4358) (-7.5328, 45.2284) knots 0 0 0 1 2 2 2
  spline S222 degree 2 poles (-7.5328, 45.2284) (-7.5328, 45.0209) (-7.3318, 44.5801) (-7.1697, 44.3694) knots 0 0 0 1 2 2 2
  line L218 (-7.1697, 44.3694) -> (-4.9266, 44.3694)
  line L219 (-4.9266, 44.3694) -> (-4.9266, 43.8151)
  line L220 (-4.9266, 43.8151) -> (-7.9282, 43.8151)
  line L221 (-7.9282, 43.8151) -> (-7.9282, 44.3694)
  line L222 (-7.9282, 44.3694) -> (-7.5943, 44.3694)
  spline S223 degree 2 poles (-7.5943, 44.3694) (-7.7986, 44.619) (-8.0125, 45.102) (-8.0125, 45.371) knots 0 0 0 1 2 2 2
  spline S224 degree 2 poles (-8.0125, 45.371) (-8.0125, 45.8572) (-7.429, 46.4083) (-6.8747, 46.4083) knots 0 0 0 1 2 2 2
  line L223 (-6.8747, 46.4083) -> (-4.9266, 46.4083)
  spline S225 degree 2 poles (-4.4469, 47.3094) (-4.4242, 47.3645) (-4.3528, 47.5849) (-4.3237, 47.7211) knots 0 0 0 1 2 2 2
  spline S226 degree 2 poles (-4.3237, 47.7211) (-4.288, 47.8767) (-4.2459, 48.136) (-4.2459, 48.2883) knots 0 0 0 1 2 2 2
  spline S227 degree 2 poles (-4.2459, 48.2883) (-4.2459, 48.5444) (-4.3691, 48.901) (-4.4793, 49.0015) knots 0 0 0 1 2 2 2
  spline S228 degree 2 poles (-4.4793, 49.0015) (-4.5895, 49.0955) (-4.878, 49.1733) (-5.0627, 49.1733) knots 0 0 0 1 2 2 2
  line L224 (-5.0627, 49.1733) -> (-5.3253, 49.1733)
  spline S229 degree 2 poles (-5.3253, 49.1733) (-5.147, 48.9496) (-4.9785, 48.5185) (-4.9785, 48.1943) knots 0 0 0 1 2 2 2
  spline S230 degree 2 poles (-4.9785, 48.1943) (-4.9785, 47.6303) (-5.7402, 46.9626) (-6.4566, 46.9626) knots 0 0 0 1 2 2 2
  spline S231 degree 2 poles (-6.4566, 46.9626) (-6.8293, 46.9626) (-7.4063, 47.1927) (-7.6105, 47.3872) knots 0 0 0 1 2 2 2
  spline S232 degree 2 poles (-7.6105, 47.3872) (-7.8018, 47.572) (-8.0125, 48.0809) (-8.0125, 48.3532) knots 0 0 0 1 2 2 2
  spline S233 degree 2 poles (-8.0125, 48.3532) (-8.0125, 48.6093) (-7.9023, 48.9853) (-7.8018, 49.1733) knots 0 0 0 1 2 2 2
  line L225 (-7.8018, 49.1733) -> (-7.9282, 49.2057)
  line L226 (-7.9282, 49.2057) -> (-7.9282, 49.7276)
  line L227 (-7.9282, 49.7276) -> (-5.2702, 49.7276)
  spline S234 degree 2 poles (-5.2702, 49.7276) (-4.5052, 49.7276) (-3.7921, 48.995) (-3.7921, 48.243) knots 0 0 0 1 2 2 2
  spline S235 degree 2 poles (-3.7921, 48.243) (-3.7921, 48.0031) (-3.8634, 47.4974) (-3.9217, 47.2802) knots 0 0 0 1 2 2 2
  line L228 (-3.9217, 47.2802) -> (-4.4469, 47.2802)
  line L229 (-4.4469, 47.2802) -> (-4.4469, 47.3094)
  line L230 (-5.7402, 49.1733) -> (-7.3901, 49.1733)
  spline S236 degree 2 poles (-7.3901, 49.1733) (-7.4809, 48.9658) (-7.5587, 48.6157) (-7.5587, 48.4407) knots 0 0 0 1 2 2 2
  spline S237 degree 2 poles (-7.5587, 48.4407) (-7.5587, 48.0193) (-6.9947, 47.5363) (-6.4663, 47.5363) knots 0 0 0 1 2 2 2
  spline S238 degree 2 poles (-6.4663, 47.5363) (-5.9671, 47.5363) (-5.4452, 47.9058) (-5.4452, 48.3175) knots 0 0 0 1 2 2 2
  spline S239 degree 2 poles (-5.4452, 48.3175) (-5.4452, 48.5347) (-5.6008, 48.9917) (-5.7402, 49.1733) knots 0 0 0 1 2 2 2
  line L231 (-4.9266, 51.0955) -> (-4.9266, 50.5412)
  line L232 (-4.9266, 50.5412) -> (-7.9282, 50.5412)
  line L233 (-7.9282, 50.5412) -> (-7.9282, 51.0955)
  line L234 (-7.9282, 51.0955) -> (-4.9266, 51.0955)
  line L235 (-8.4274, 51.1376) -> (-8.4274, 50.5055)
  line L236 (-8.4274, 50.5055) -> (-8.9525, 50.5055)
  line L237 (-8.9525, 50.5055) -> (-8.9525, 51.1376)
  line L238 (-8.9525, 51.1376) -> (-8.4274, 51.1376)
  line L239 (-4.9266, 54.5055) -> (-4.9266, 53.9512)
  line L240 (-4.9266, 53.9512) -> (-6.6381, 53.9512)
  spline S240 degree 2 poles (-6.6381, 53.9512) (-6.8456, 53.9512) (-7.2021, 53.9058) (-7.3091, 53.8443) knots 0 0 0 1 2 2 2
  spline S241 degree 2 poles (-7.3091, 53.8443) (-7.4225, 53.7762) (-7.5328, 53.5331) (-7.5328, 53.3256) knots 0 0 0 1 2 2 2
  spline S242 degree 2 poles (-7.5328, 53.3256) (-7.5328, 53.1182) (-7.3318, 52.6773) (-7.1697, 52.4666) knots 0 0 0 1 2 2 2
  line L241 (-7.1697, 52.4666) -> (-4.9266, 52.4666)
  line L242 (-4.9266, 52.4666) -> (-4.9266, 51.9123)
  line L243 (-4.9266, 51.9123) -> (-7.9282, 51.9123)
  line L244 (-7.9282, 51.9123) -> (-7.9282, 52.4666)
  line L245 (-7.9282, 52.4666) -> (-7.5943, 52.4666)
  spline S243 degree 2 poles (-7.5943, 52.4666) (-7.7986, 52.7162) (-8.0125, 53.1992) (-8.0125, 53.4682) knots 0 0 0 1 2 2 2
  spline S244 degree 2 poles (-8.0125, 53.4682) (-8.0125, 53.9545) (-7.429, 54.5055) (-6.8747, 54.5055) knots 0 0 0 1 2 2 2
  line L246 (-6.8747, 54.5055) -> (-4.9266, 54.5055)
  spline S245 degree 2 poles (-4.8585, 56.7195) (-4.8585, 55.9318) (-5.6657, 55.0598) (-6.4112, 55.0598) knots 0 0 0 1 2 2 2